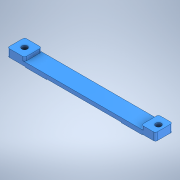
# Autodesk Inventor part: HullMid
Saved by Autodesk Inventor 2021 (Build 250183000, 183)
## iProperties
Created: 2021-05-14
Part Number: HullMid
Material: Generic
Document SubType Name: Modeling
Designer: ermoz
Density: 1 g/cm^3
Appearance: Default
Author: ermoz
Autodesk Inventor part; units mm, degrees
ref_plane "YZ Plane" through (0, 0, 0) normal (1, 0, 0) x (0, 1, 0)
ref_plane "XZ Plane" through (0, 0, 0) normal (0, 1, 0) x (-1, 0, 0)
ref_plane "XY Plane" through (0, 0, 0) normal (0, 0, 1) x (1, 0, 0)
sketch "Sketch1" plane through (0, 0, 0) normal (0, 1, 0) x (-1, 0, 0)
  line L0 (0, 0) -> (77.6, 0)
  line L1 (77.6, 0) -> (77.6, -9)
  line L2 (77.6, -9) -> (0, -9)
  line L3 (0, -9) -> (0, 0)
  line L4 (50.291, 0) -> (28.6614, 0)
  line L5 (77.6, -9) -> (68.6, -9)
  line L6 (68.6, -9) -> (68.6, 0)
  line L7 (68.6, 0) -> (77.6, 0)
  line L8 (77.6, 0) -> (77.6, -9)
  line L9 (68.6, -9) -> (56.6, -9)
  line L10 (56.6, -9) -> (56.6, 0)
  line L11 (56.6, 0) -> (68.6, 0)
  line L12 (68.6, 0) -> (68.6, -9)
  line L13 (18.6, -9) -> (6.6, -9)
  line L14 (6.6, -9) -> (6.6, 0)
  line L15 (6.6, 0) -> (18.6, 0)
  line L16 (18.6, 0) -> (18.6, -9)
  line L17 (68.6, -9) -> (56.6, -9)
  line L18 (18.6, -9) -> (6.6, -9)
  line L19 (68.6, -9) -> (56.6, -9)
  line L20 (56.6, -9) -> (56.6, 0)
  line L21 (56.6, 0) -> (68.6, 0)
  line L22 (68.6, 0) -> (68.6, -9)
  line L23 (68.6, -9) -> (56.6, 0) construction
  line L24 (56.6, -9) -> (68.6, 0) construction
  line L25 (6.6, -9) -> (18.6, -9)
  line L26 (18.6, -9) -> (18.6, 0)
  line L27 (18.6, 0) -> (6.6, 0)
  line L28 (6.6, 0) -> (6.6, -9)
  line L29 (6.6, -9) -> (18.6, 0) construction
  line L30 (18.6, -9) -> (6.6, 0) construction
  line L31 (62.6, 0) -> (12.6, 0)
  line L32 (12.6, 0) -> (12.6, 15)
  line L33 (12.6, 15) -> (62.6, 15)
  line L34 (62.6, 15) -> (62.6, 0)
  point P0 (62.6, -4.5)
  point P1 (12.6, -4.5)
  point P2 (62.6, 0)
  point P3 (12.6, 0)
  point P4 (12.6, -4.5)
  dimension "d0" = 77.6
  dimension "d1" = 9
  dimension "d3" = 9
  dimension "d4" = 12
  dimension "d5" = 12
  dimension "d6" = 50
  dimension "d7" = 15
  constraints: 70 end point, 14 parallel, 8 horizontal, 7 perpendicular, 6 midpoint, 5 point on line, 2 collinear
  measures "d0" distance of L1.end L2.end
  measures "d1" distance of L0.end L1.end
  measures "d3" distance of L6.end L7.end
  measures "d4" distance of L10.end L11.end
  measures "d5" distance of L14.end L15.end
  measures "d6" distance of point (12.6, -4.5) point (62.6, -4.5)
  measures "d7" distance of L31.end L32.end
extrude "Extrusion1" add sketch "Sketch1" along normal blind 13.5
sketch "Sketch2" plane through (-62.6, 0, 15) normal (0, 0, 1) x (1, 0, 0)
  line L0 (0, 0) -> (0, 13.5) projected
  circle A0 centre (0, 0) radius 14.5
  line L1 (50, 0) -> (50, 13.5) projected
  circle A1 centre (50, 0) radius 14.5
  circle A2 centre (0, 0) radius 16.5
  circle A3 centre (50, 0) radius 16.5
  line L2 (6, -5) -> (-6, -5)
  line L3 (-6, -5) -> (-6, 5)
  line L4 (-6, 5) -> (6, 5)
  line L5 (6, 5) -> (6, -5)
  line L6 (6, -5) -> (-6, 5) construction
  line L7 (-6, -5) -> (6, 5) construction
  line L8 (56, -5) -> (44, -5)
  line L9 (44, -5) -> (44, 5)
  line L10 (44, 5) -> (56, 5)
  line L11 (56, 5) -> (56, -5)
  line L12 (56, -5) -> (44, 5) construction
  line L13 (44, -5) -> (56, 5) construction
  line L14 (56, 5) -> (73.1985, 5)
  line L15 (62.6, 0) -> (62.6, 13.5) projected
  line L16 (44, 5) -> (35, 5)
  line L17 (35, 5) -> (35, 0)
  line L18 (35, 0) -> (15, 0)
  line L19 (62.6, 0) -> (-15, 0) projected
  line L20 (15, 5) -> (6, 5)
  line L21 (15, 5) -> (15, 0)
  line L22 (-6, 5) -> (-20.1894, 5)
  point P0 (-15.7242, 5)
  point P1 (16.5, 0)
  point P2 (6, 0)
  point P3 (-6, 0)
  point P4 (62.6, 5)
  dimension "d10" = 29
  dimension "d11" = 29
  dimension "d12" = 2
  dimension "d13" = 2
  dimension "d14" = 12
  dimension "d15" = 10
  dimension "d16" = 12
  dimension "d17" = 10
  dimension "d18" = 9
  dimension "d19" = 9
  constraints: 38 end point, 5 parallel, 5 perpendicular, 4 centre point, 4 horizontal, 4 midpoint, 2 point on line
  measures "d10" diameter of A0
  measures "d11" diameter of A1
  measures "d12" radial gap between concentric circles of A0 A2
  measures "d13" radial gap between concentric circles of A1 A3
  measures "d14" distance of L3.end L4.end
  measures "d15" distance of L2.end L3.end
  measures "d16" distance of L9.end L10.end
  measures "d17" distance of L8.end L9.end
  measures "d18" distance of L20.start L4.end
  measures "d19" distance of L9.end L16.end
extrude "Extrusion2" cut sketch "Sketch2" against normal up to surface (15 mm away)
extrude "Extrusion3" cut sketch "Sketch2" against normal through all contours L19 L3 L4 L0 | L0 L4 L5 L19 | L19 A0 L3 L2 L5 | L5 L20 A0 L19 | L19 A0 L22 L3 | L19 L18 A2 L22 A0 | A0 L20 L21 L19 | L19 L9 L10 L1 | L1 L10 L11 L19 | L11 L14 L15 L19 | L19 A1 L16 L9 | L19 L17 L16 A1
sketch "Sketch3" plane through (0, 13.5, -9) normal (0, 0, -1) x (-1, 0, 0)
  line L0 (27.6, -8.5) -> (27.6, -13.5) projected
  line L1 (47.6, -8.5) -> (47.6, -13.5) projected
  line L2 (27.6, -8.5) -> (47.6, -8.5)
  line L3 (47.6, -8.5) -> (47.6, -13.5)
  line L4 (47.6, -13.5) -> (27.6, -13.5)
  line L5 (27.6, -13.5) -> (27.6, -8.5)
  point P0 (0, -13.5)
  constraints: 8 end point, 2 parallel, 1 horizontal, 1 perpendicular
extrude "Extrusion4" cut sketch "Sketch3" against normal blind 4
sketch "Sketch4" plane through (0, 13.5, 0) normal (0, 1, 0) x (1, 0, 0)
  circle A0 centre (-73.1, 4.5) radius 1.5
  line L0 (-77.6, 9) -> (-77.6, 0) projected
  circle A1 centre (-2.9, 4.5) radius 1.5
  line L1 (0, 0) -> (0, 9) projected
  point P0 (-77.6, 4.5)
  dimension "d26" = 3
  dimension "d27" = 4.5
  dimension "d45" = 3
  dimension "d46" = 2.9
  constraints: 2 centre point, 1 horizontal alignment, 1 midpoint
  measures "d26" diameter of A0
  measures "d27" distance from line of L0 A0.centre
  measures "d45" diameter of A1
  measures "d46" distance from line of L1 A1.centre
extrude "Extrusion5" cut sketch "Sketch4" against normal through all
sketch "Sketch5" plane through (0, 13.5, 0) normal (0, 1, 0) x (1, 0, 0)
  line L0 (-77.6, 9) -> (-77.6, 0) projected
  line L1 (-77.6, 0) -> (0, 0) projected
  line L2 (-77.6, 9) -> (0, 9)
  line L3 (0, 9) -> (0, 0)
  line L4 (0, 0) -> (-77.6, 0)
  line L5 (-77.6, 0) -> (-77.6, 9)
  circle A0 centre (-3, 4.5) radius 1.5
  point P0 (-28.5, 0)
  dimension "d43" = 3
  dimension "d44" = 3
  constraints: 8 end point, 2 parallel, 1 centre point, 1 horizontal, 1 perpendicular
  measures "d43" diameter of A0
  measures "d44" distance from line of L3 A0.centre
extrude "Extrusion6" cut sketch "Sketch5" against normal blind 4.5 contours L2 L3 L1 L0 | A0
sketch "Sketch6" plane through (0, 5, -9) normal (0, 0, -1) x (-1, 0, 0)
  line L0 (77.6, 0) -> (47.6, 0) projected
  line L1 (77.6, 0) -> (77.6, 4) projected
  line L2 (0, 0) -> (77.6, 0)
  line L3 (77.6, 0) -> (77.6, 2)
  line L4 (77.6, 2) -> (0, 2)
  line L5 (0, 2) -> (0, 0)
  point P0 (0, -5)
  point P1 (28.5, 0)
  point P2 (77.6, 0)
  dimension "d32" = 2
  constraints: 8 end point, 2 parallel, 1 horizontal, 1 midpoint, 1 perpendicular
  measures "d32" distance between parallel lines of L4 L2
extrude "Extrusion7" add sketch "Sketch6" along normal blind 5
sketch "Sketch8" plane through (-77.6, 7, -9) normal (0, 1, 0) x (1, 0, 0)
  line L0 (77.6, 5) -> (0, 5) projected
  line L1 (0, 0) -> (77.6, 0) projected
  line L2 (0, 5) -> (10, 5)
  line L3 (10, 5) -> (10, 0)
  line L4 (10, 0) -> (0, 0)
  line L5 (0, 0) -> (0, 5)
  point P0 (77.6, -9)
  point P1 (74.6, 0)
  dimension "d38" = 10
  constraints: 8 end point, 2 parallel, 1 horizontal, 1 perpendicular, 1 point on line
  measures "d38" distance between parallel lines of L5 L3
extrude "Extrusion9" cut sketch "Sketch8" against normal through all
fillet "Fillet1" radius 1 8 edges at (-53.1132, 13.5, 7.5) (-22.0868, 13.5, 7.5) (-67.6, 6, -9) (-67.6, 6, -14) (0, 6, -14) (0, 7, 0) (-77.6, 7, 0) (-77.6, 7, -9)
sketch "Sketch9" plane through (-46.1, 0, 15) normal (0, 0, 1) x (1, 0, 0)
  line L0 (-16.4583, 22.1349) -> (30.9357, 22.1349)
  line L1 (30.9357, 22.1349) -> (30.9357, -8.4055)
  line L2 (30.9357, -8.4055) -> (-16.4583, -8.4055)
  line L3 (-16.4583, -8.4055) -> (-16.4583, 22.1349)
  point P0 (46.1, 0)
  constraints: 8 end point, 2 parallel, 1 horizontal, 1 perpendicular
extrude "Extrusion10" cut sketch "Sketch9" against normal up to surface (15 mm away)
sketch "Sketch10" plane through (0, 0, 0) normal (0, -1, 0) x (1, 0, 0)
  line L0 (-27.6, 0) -> (-27.6, -5) projected
  line L1 (-47.6, 0) -> (-47.6, -5) projected
  line L2 (-27.6, 0) -> (-47.6, 0)
  line L3 (-47.6, 0) -> (-47.6, -5)
  line L4 (-47.6, -5) -> (-27.6, -5)
  line L5 (-27.6, -5) -> (-27.6, 0)
  point P0 (0, 0)
  constraints: 8 end point, 2 parallel, 1 horizontal, 1 perpendicular
extrude "Extrusion11" cut sketch "Sketch10" against normal up to surface (5 mm away)
sketch "Sketch11" plane through (0, 9, 0) normal (0, 1, 0) x (1, 0, 0)
  line L0 (1.6, 0) -> (-7.4, 0)
  line L1 (-7.4, 0) -> (-7.4, 9)
  line L2 (-7.4, 9) -> (1.6, 9)
  line L3 (1.6, 9) -> (1.6, 0)
  circle A0 centre (-2.9, 4.5) radius 1.5 projected
  line L4 (1.6, 0) -> (-7.4, 9) construction
  line L5 (-7.4, 0) -> (1.6, 9) construction
  line L6 (0, 9) -> (-68.6, 9) projected
  line L7 (-77.6, 0) -> (-68.6, 0)
  line L8 (-68.6, 0) -> (-68.6, 9)
  line L9 (-68.6, 9) -> (-77.6, 9)
  line L10 (-77.6, 9) -> (-77.6, 0)
  circle A1 centre (-73.1, 4.5) radius 1.5 projected
  line L11 (-77.6, 0) -> (-68.6, 9) construction
  line L12 (-68.6, 0) -> (-77.6, 9) construction
  arc A2 (-68.6, 9) -> (-67.6, 10) centre (-68.6, 10) ccw projected
  line L13 (-7.4, 0) -> (-68.6, 0)
  line L14 (-68.6, 0) -> (-68.6, 9)
  line L15 (-68.6, 9) -> (-7.4, 9)
  line L16 (-7.4, 9) -> (-7.4, 0)
  point P0 (0, 0)
  point P1 (-4, 9)
  dimension "d51" = 9
  dimension "d52" = 9
  dimension "d53" = 9
  dimension "d54" = 9
  constraints: 32 end point, 6 parallel, 4 midpoint, 3 horizontal, 3 perpendicular
  measures "d51" distance of L1.end L2.end
  measures "d52" distance of L0.end L1.end
  measures "d53" distance of L9.end L6.end
  measures "d54" distance of L6.end L7.end
extrude "Extrusion12" cut sketch "Sketch11" against normal up to surface (2 mm away) contours L13 L8 L6 L1
fillet "Fillet3" radius 1 5 edges at (-68.6, 8, -9) (-68.6, 8, 0) (-7.4, 8, -9) (-7.4, 8, 0) (0, 8, -9)
sketch "Sketch12" plane through (-66.6, 7, -14) normal (0, 1, 0) x (1, 0, 0)
  line L0 (-3.8589, -5) -> (66.6, -5)
  line L1 (66.6, -5) -> (66.6, 0)
  line L2 (66.6, 0) -> (-3.8589, 0)
  line L3 (-3.8589, 0) -> (-3.8589, -5)
  point P0 (66.6, -14)
  constraints: 8 end point, 2 parallel, 1 horizontal, 1 perpendicular
extrude "Extrusion13" cut sketch "Sketch12" against normal through all
fillet "Fillet4" radius 1 1 edges at (0, 6, -9)
sketch "Sketch13" plane through (-76.6, 5, 0) normal (0, -1, 0) x (1, 0, 0)
  line L0 (8.5, 0) -> (19.5, 0)
  line L1 (19.5, 0) -> (19.5, -9)
  line L2 (19.5, -9) -> (8.5, -9)
  line L3 (8.5, -9) -> (8.5, 0)
  line L4 (58.6, 0) -> (69.6, 0)
  line L5 (69.6, 0) -> (69.6, -9)
  line L6 (69.6, -9) -> (58.6, -9)
  line L7 (58.6, -9) -> (58.6, 0)
  line L8 (0, 0) -> (75.6, 0) projected
  line L9 (0, -9) -> (75.6, -9) projected
  line L10 (-1, -8) -> (-1, -1) projected
  line L11 (76.6, -1) -> (76.6, -8) projected
  point P0 (76.6, 0)
  dimension "d61" = 9.5
  dimension "d62" = 11
  dimension "d63" = 7
  constraints: 16 end point, 5 collinear, 4 parallel, 2 horizontal, 2 perpendicular
  measures "d61" distance between parallel lines of L10 L3
  measures "d62" distance between parallel lines of L3 L1
  measures "d63" distance between parallel lines of L11 L5
extrude "Extrusion14" add sketch "Sketch13" along normal blind 0.3 contours L0 L1 L2 L3 | L4 L5 L6 L7
body "Solid1"
